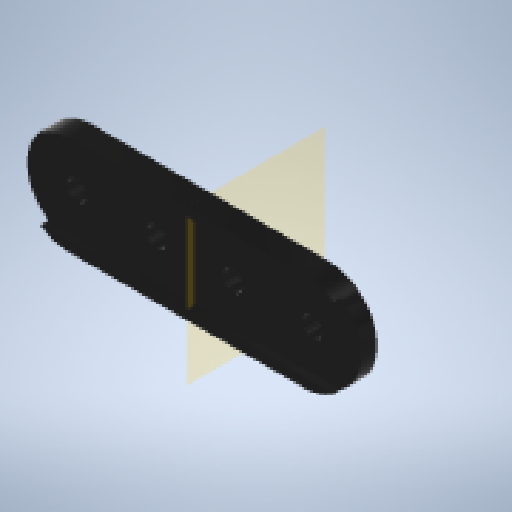
# Autodesk Inventor part: Espaciador Actuador - Antenas
Saved by Autodesk Inventor 2024.2 (Build 282272000, 272)
## iProperties
Created: 2023-12-10
Part Number: Espaciador Actuador - Antenas
Material: PET Plastic
Document SubType Name: Modeling
Designer: juanp
Density: 1.541 g/cm^3
Appearance: Smooth - Black
Author: juanp
Autodesk Inventor part; units mm, degrees
ref_plane "YZ Plane" through (0, 0, 0) normal (1, 0, 0) x (0, 1, 0)
ref_plane "XZ Plane" through (0, 0, 0) normal (0, 1, 0) x (-1, 0, 0)
ref_plane "XY Plane" through (0, 0, 0) normal (0, 0, 1) x (1, 0, 0)
sketch "Sketch1" plane through (0, 0, 0) normal (0, 0, 1) x (1, 0, 0)
  arc A0 (-3, 3) -> (0, 0) centre (0, 3) ccw construction
  line L0 (0, 0) -> (121, 0) construction
  arc A1 (121, 0) -> (124, 3) centre (121, 3) ccw construction
  line L1 (124, 3) -> (124, 85) construction
  arc A2 (124, 85) -> (121, 88) centre (121, 85) ccw construction
  line L2 (121, 88) -> (0, 88) construction
  arc A3 (0, 88) -> (-3, 85) centre (0, 85) ccw construction
  line L3 (-3, 85) -> (-3, 3) construction
  arc A4 (63.75, 4.5) -> (63.75, 7.5) centre (63.75, 6) ccw construction
  line L4 (57.25, 4.5) -> (63.75, 4.5) construction
  arc A5 (57.25, 7.5) -> (57.25, 4.5) centre (57.25, 6) ccw construction
  line L5 (63.75, 7.5) -> (57.25, 7.5) construction
  arc A6 (70.5, 11.18) -> (70.5, 16.18) centre (70.5, 13.68) ccw construction
  line L6 (50.5, 11.18) -> (70.5, 11.18) construction
  arc A7 (50.5, 16.18) -> (50.5, 11.18) centre (50.5, 13.68) ccw construction
  line L7 (70.5, 16.18) -> (50.5, 16.18) construction
  arc A8 (43.75, 80.5) -> (43.75, 83.5) centre (43.75, 82) ccw construction
  line L8 (37.25, 80.5) -> (43.75, 80.5) construction
  arc A9 (37.25, 83.5) -> (37.25, 80.5) centre (37.25, 82) ccw construction
  line L9 (43.75, 83.5) -> (37.25, 83.5) construction
  arc A10 (70.5, 71.82) -> (70.5, 76.82) centre (70.5, 74.32) ccw construction
  line L10 (50.5, 71.82) -> (70.5, 71.82) construction
  arc A11 (50.5, 76.82) -> (50.5, 71.82) centre (50.5, 74.32) ccw construction
  line L11 (70.5, 76.82) -> (50.5, 76.82) construction
  circle A12 centre (30.65, 13.68) radius 3.55 construction
  circle A13 centre (10.65, 23.68) radius 2.55 construction
  circle A14 centre (30.65, 23.68) radius 2.55
  circle A15 centre (50.81, 23.68) radius 2.55
  circle A16 centre (80.35, 23.68) radius 2.55 construction
  circle A17 centre (100.35, 23.68) radius 2.55 construction
  circle A18 centre (100.35, 13.68) radius 2.55 construction
  circle A19 centre (80.35, 44) radius 2.55 construction
  circle A20 centre (90.35, 44) radius 2.55 construction
  circle A21 centre (80.35, 13.68) radius 2.55 construction
  circle A22 centre (100.35, 64.32) radius 2.55 construction
  circle A23 centre (80.35, 74.32) radius 2.55 construction
  circle A24 centre (90.35, 74.32) radius 2.55 construction
  circle A25 centre (30.65, 74.32) radius 3.55 construction
  circle A26 centre (40.18, 34) radius 2.55 construction
  circle A27 centre (30.65, 44) radius 3.55 construction
  circle A28 centre (70.19, 64.32) radius 2.55 construction
  circle A29 centre (20.65, 44) radius 3.55 construction
  circle A30 centre (60.5, 34) radius 2.55 construction
  circle A31 centre (100.35, 74.32) radius 2.55 construction
  circle A32 centre (90.82, 34) radius 2.55 construction
  circle A33 centre (110.35, 74.32) radius 2.55 construction
  circle A34 centre (90.82, 54) radius 2.55 construction
  circle A35 centre (75.325, 58.825) radius 2.55 construction
  circle A36 centre (30.65, 64.32) radius 2.55 construction
  circle A37 centre (10.65, 64.32) radius 2.55 construction
  circle A38 centre (45.675, 58.825) radius 2.55 construction
  circle A39 centre (10.65, 13.68) radius 3.55 construction
  circle A40 centre (10.65, 74.32) radius 3.55 construction
  circle A41 centre (50.5, 44) radius 2.55 construction
  circle A42 centre (60.5, 54) radius 2.55 construction
  circle A43 centre (60.5, 44) radius 2.55 construction
  circle A44 centre (70.5, 44) radius 2.55 construction
  circle A45 centre (40.18, 54) radius 2.55 construction
  circle A46 centre (10.65, 44) radius 3.55 construction
  circle A47 centre (30.18, 54) radius 2.55 construction
  circle A48 centre (60.5, 64.32) radius 2.55 construction
  circle A49 centre (20.65, 64.32) radius 2.55 construction
  circle A50 centre (20.65, 74.32) radius 3.55 construction
  circle A51 centre (80.82, 54) radius 2.55 construction
  circle A52 centre (40.65, 64.32) radius 2.55 construction
  circle A53 centre (110.35, 44) radius 2.55 construction
  circle A54 centre (110.35, 13.68) radius 2.55 construction
  circle A55 centre (80.82, 34) radius 2.55 construction
  circle A56 centre (75.325, 29.175) radius 2.55 construction
  circle A57 centre (50.81, 64.32) radius 2.55 construction
  circle A58 centre (80.35, 64.32) radius 2.55 construction
  circle A59 centre (45.675, 29.175) radius 2.55 construction
  circle A60 centre (30.18, 34) radius 2.55 construction
  circle A61 centre (40.65, 74.32) radius 3.55 construction
  circle A62 centre (40.65, 44) radius 3.55 construction
  circle A63 centre (90.35, 64.32) radius 2.55 construction
  circle A64 centre (110.35, 64.32) radius 2.55 construction
  circle A65 centre (100.35, 44) radius 2.55 construction
  circle A66 centre (60.5, 23.68) radius 2.55 construction
  circle A67 centre (90.35, 13.68) radius 2.55 construction
  circle A68 centre (110.35, 23.68) radius 2.55 construction
  circle A69 centre (90.35, 23.68) radius 2.55
  circle A70 centre (70.19, 23.68) radius 2.55
  circle A71 centre (40.65, 23.68) radius 2.55 construction
  circle A72 centre (20.65, 23.68) radius 2.55 construction
  circle A73 centre (40.65, 13.68) radius 3.55 construction
  circle A74 centre (20.65, 13.68) radius 3.55 construction
  arc A75 (63.75, 80.5) -> (63.75, 83.5) centre (63.75, 82) ccw construction
  line L12 (57.25, 80.5) -> (63.75, 80.5) construction
  arc A76 (57.25, 83.5) -> (57.25, 80.5) centre (57.25, 82) ccw construction
  line L13 (63.75, 83.5) -> (57.25, 83.5) construction
  arc A77 (77.25, 83.5) -> (77.25, 80.5) centre (77.25, 82) ccw construction
  line L14 (83.75, 83.5) -> (77.25, 83.5) construction
  arc A78 (83.75, 80.5) -> (83.75, 83.5) centre (83.75, 82) ccw construction
  line L15 (77.25, 80.5) -> (83.75, 80.5) construction
  arc A79 (43.75, 4.5) -> (43.75, 7.5) centre (43.75, 6) ccw construction
  line L16 (37.25, 4.5) -> (43.75, 4.5) construction
  arc A80 (37.25, 7.5) -> (37.25, 4.5) centre (37.25, 6) ccw construction
  line L17 (43.75, 7.5) -> (37.25, 7.5) construction
  arc A81 (77.25, 7.5) -> (77.25, 4.5) centre (77.25, 6) ccw construction
  line L18 (83.75, 7.5) -> (77.25, 7.5) construction
  arc A82 (83.75, 4.5) -> (83.75, 7.5) centre (83.75, 6) ccw construction
  line L19 (77.25, 4.5) -> (83.75, 4.5) construction
  line L20 (30.65, 23.68) -> (90.35, 23.68) construction
  line L21 (30.65, 11.18) -> (90.35, 11.18)
  line L22 (90.35, 36.18) -> (30.65, 36.18)
  arc A83 (30.65, 36.18) -> (30.65, 11.18) centre (30.65, 23.68) ccw
  arc A84 (90.35, 11.18) -> (90.35, 36.18) centre (90.35, 23.68) ccw
  line L23 (23.3543, 33.83) -> (97.6457, 33.83)
  line L24 (23.3543, 13.53) -> (97.6457, 13.53)
  point P0 (60.5, 23.68)
  dimension "d0" = 25
  dimension "d3" = 20.3
  constraints: 85 centre point, 52 end point, 48 point on circle, 20 horizontal, 4 tangent, 3 parallel, 2 vertical, 1 midpoint, 207 other
  measures "d0" distance between parallel lines of L22 L21
  measures "d3" distance between parallel lines of L24 L23
extrude "Extrusion1" add sketch "Sketch1" along normal blind 4
extrude "Extrusion2" add sketch "Sketch1" along normal blind 6 contours A83 L24 A84 L21 | A83 L22 A84 L23
sketch "Sketch2" plane through (30.65, 36.18, 0) normal (0, 1, 0) x (1, 0, 0)
  line L0 (0, -6) -> (59.7, -6) projected
  line L1 (29.85, -6) -> (29.85, 29.1247)
  point P0 (-30.65, 0)
  constraints: 2 end point, 1 midpoint, 1 vertical
surface extrude "ExtrusionSrf1" sketch "Sketch2" against normal blind 39.35 shown yes curves L1
body "Solid1"
body "Srf1"
